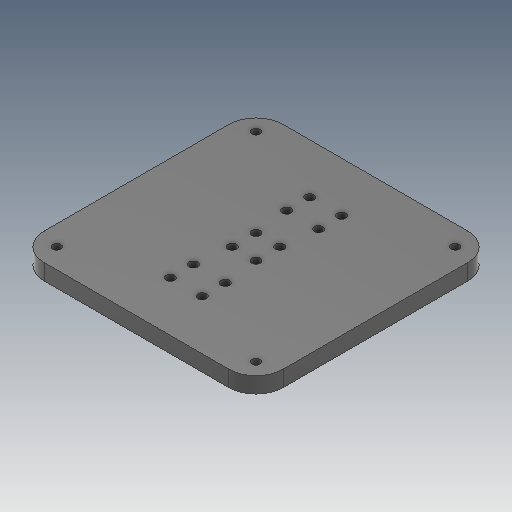
# Autodesk Inventor part: VerticalActuationMount
Saved by Autodesk Inventor 2020.3 (Build 243373000, 373)
## iProperties
Created: 2021-09-01
Part Number: VerticalActuationMount
Material: ABS Plastic
Document SubType Name: Modeling
Designer: justi
Density: 1.06 g/cm^3
Appearance: Smooth - Black
Mass: 229.675 g
Surface Area: 526.889 cm^2
Volume: 216.675 cm^3
Author: justi
Autodesk Inventor part; units mm, degrees
ref_plane "YZ Plane" through (0, 0, 0) normal (1, 0, 0) x (0, 1, 0)
ref_plane "XZ Plane" through (0, 0, 0) normal (0, 1, 0) x (-1, 0, 0)
ref_plane "XY Plane" through (0, 0, 0) normal (0, 0, 1) x (1, 0, 0)
sketch "Sketch1" plane through (0, 0, 0) normal (0, 1, 0) x (-1, 0, 0)
  line L0 (75, 75) -> (-75, 75)
  line L1 (-75, 75) -> (-75, -75)
  line L2 (-75, -75) -> (75, -75)
  line L3 (75, -75) -> (75, 75)
  line L4 (75, 75) -> (-75, -75) construction
  line L5 (-75, 75) -> (75, -75) construction
  point P0 (0, 0)
  dimension "d0" = 150
  dimension "d1" = 150
  constraints: 12 end point, 2 midpoint, 2 parallel, 1 horizontal, 1 perpendicular
  measures "d0" distance of L2.end L1.end
  measures "d1" distance of L1.end L0.end
extrude "Extrusion1" add sketch "Sketch1" along normal blind 10
sketch "Sketch2" plane through (0, 10, 0) normal (0, 1, 0) x (1, 0, 0)
  line L0 (-10, 43.75) -> (10, 43.75)
  line L1 (10, 43.75) -> (10, -43.75)
  line L2 (10, -43.75) -> (-10, -43.75)
  line L3 (-10, -43.75) -> (-10, 43.75)
  line L4 (-10, -29.25) -> (10, -29.25)
  line L5 (10, -29.25) -> (10, 29.25)
  line L6 (10, 29.25) -> (-10, 29.25)
  line L7 (-10, 29.25) -> (-10, -29.25)
  circle A0 centre (-10, 43.75) radius 2.5
  circle A1 centre (10, 43.75) radius 2.5
  circle A2 centre (-10, 29.25) radius 2.5
  circle A3 centre (10, 29.25) radius 2.5
  circle A4 centre (10, -29.25) radius 2.5
  circle A5 centre (-10, -29.25) radius 2.5
  circle A6 centre (-10, -43.75) radius 2.5
  circle A7 centre (10, -43.75) radius 2.5
  line L8 (-75, 75) -> (-75, -75) projected
  point P0 (0, 0)
  dimension "d4" = 20
  dimension "d5" = 87.5
  dimension "d6" = 58.5
  dimension "d7" = 5
  dimension "d8" = 5
  dimension "d9" = 5
  dimension "d10" = 5
  dimension "d11" = 5
  dimension "d12" = 5
  dimension "d13" = 5
  dimension "d14" = 5
  dimension "d51" = 75
  constraints: 16 end point, 8 centre point, 8 coincident, 4 parallel, 2 horizontal, 2 perpendicular, 1 point on line
  measures "d4" distance of L1.end L2.end
  measures "d5" distance of L0.end L1.end
  measures "d6" distance of L5.end L4.end
  measures "d7" diameter of A0
  measures "d8" diameter of A1
  measures "d9" diameter of A2
  measures "d10" diameter of A3
  measures "d11" diameter of A4
  measures "d12" diameter of A5
  measures "d13" diameter of A6
  measures "d14" diameter of A7
  measures "d51" distance from line of L8 point (0, 0)
extrude "Extrusion2" cut sketch "Sketch2" against normal through all contours L3 A0 L0 | L0 A0 L3 | A1 L1 L0 | L0 L1 A1 | A2 L6 L3 | L3 A2 | L6 A2 L3 | A3 L1 | L1 L6 A3 | L6 L1 A3 | A5 L4 L3 | L3 A5 | L4 A5 L3 | A4 L1 | L1 L4 A4 | L4 L1 A4 | A6 L2 L3 | L3 L2 A6 | A7 L2 L1 | L1 L2 A7
fillet "Fillet1" radius 17 4 edges at (75, 5, 75) (-75, 5, 75) (75, 5, -75) (-75, 5, -75)
sketch "Sketch5" plane through (0, 0, 0) normal (0, -1, 0) x (1, 0, 0)
  circle A0 centre (-10, 43.75) radius 2.5 projected
  circle A1 centre (10, 43.75) radius 2.5 projected
  circle A2 centre (-10, 29.25) radius 2.5 projected
  circle A3 centre (10, 29.25) radius 2.5 projected
  circle A4 centre (-10, -29.25) radius 2.5 projected
  circle A5 centre (10, -29.25) radius 2.5 projected
  circle A6 centre (-10, -43.75) radius 2.5 projected
  circle A7 centre (10, -43.75) radius 2.5 projected
  point P0 (0, 0)
  constraints: 8 coincident
hole "Hole2" at (-10, 0, 43.75) at (10, 0, 43.75) at (-10, 0, 29.25) at (10, 0, 29.25) at (-10, 0, -29.25) at (10, 0, -29.25) at (-10, 0, -43.75) at (10, 0, -43.75) direction (0, 1, 0) diameter 5.5 end through all counterbore diameter 12 counterbore depth 3
sketch "Sketch6" plane through (0, 10, 0) normal (0, 1, 0) x (1, 0, 0)
  line L0 (62.5, 62.5) -> (-62.5, 62.5) construction
  line L1 (-62.5, 62.5) -> (-62.5, -62.5) construction
  line L2 (-62.5, -62.5) -> (62.5, -62.5) construction
  line L3 (62.5, -62.5) -> (62.5, 62.5) construction
  line L4 (62.5, 62.5) -> (-62.5, -62.5) construction
  line L5 (-62.5, 62.5) -> (62.5, -62.5) construction
  point P0 (0, 0)
  dimension "d80" = 125
  dimension "d81" = 125
  constraints: 12 end point, 2 midpoint, 2 parallel, 1 horizontal, 1 perpendicular
  measures "d80" distance of L2.end L1.end
  measures "d81" distance of L2.end L0.start
hole "Hole3" at (62.5, 10, -62.5) at (62.5, 10, 62.5) at (-62.5, 10, -62.5) at (-62.5, 10, 62.5) direction (0, -1, 0) diameter 5.2 end through all
sketch "Sketch7" plane through (0, 10, 0) normal (0, 1, 0) x (1, 0, 0)
  line L0 (7.5, -7.5) -> (-7.5, -7.5) construction
  line L1 (-7.5, -7.5) -> (-7.5, 7.5) construction
  line L2 (-7.5, 7.5) -> (7.5, 7.5) construction
  line L3 (7.5, 7.5) -> (7.5, -7.5) construction
  line L4 (7.5, -7.5) -> (-7.5, 7.5) construction
  line L5 (-7.5, -7.5) -> (7.5, 7.5) construction
  circle A0 centre (7.5, -7.5) radius 2.75
  circle A1 centre (-7.5, -7.5) radius 2.75
  circle A2 centre (7.5, 7.5) radius 2.75
  circle A3 centre (-7.5, 7.5) radius 2.75
  point P0 (0, 0)
  dimension "d89" = 15
  dimension "d90" = 15
  dimension "d91" = 5.5
  dimension "d92" = 5.5
  dimension "d93" = 5.5
  dimension "d94" = 5.5
  constraints: 12 end point, 4 centre point, 4 coincident, 2 midpoint, 2 parallel, 1 horizontal, 1 perpendicular
  measures "d89" distance of L1.end L2.end
  measures "d90" distance of L0.end L1.end
  measures "d91" diameter of A0
  measures "d92" diameter of A1
  measures "d93" diameter of A2
  measures "d94" diameter of A3
extrude "Extrusion4" cut sketch "Sketch7" against normal through all
equation "\"d91\" = d94"
equation "\"d92\" = d94"
equation "\"d93\" = d94"
body "Solid1"
